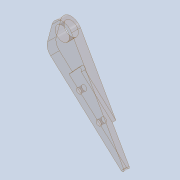
# Autodesk Inventor part: アーム先端
Saved by Autodesk Inventor 2020.4 (Build 244396000, 396)
## iProperties
Created: 2021-05-06
Part Number: アーム先端
Material: ポリカーボネート、スモーク
Document SubType Name: Modeling
Designer: happy
Density: 1.2 g/cm^3
Appearance: ポリカーボネート - スモーク
Author: happy
Autodesk Inventor part; units mm, degrees
ref_plane "YZ Plane" through (0, 0, 0) normal (1, 0, 0) x (0, 1, 0)
ref_plane "XZ Plane" through (0, 0, 0) normal (0, 1, 0) x (-1, 0, 0)
ref_plane "XY Plane" through (0, 0, 0) normal (0, 0, 1) x (1, 0, 0)
sketch "スケッチ1" plane through (0, 0, 0) normal (0, 0, 1) x (1, 0, 0)
  circle A0 centre (295.8489, -93.1201) radius 1.5
  circle A1 centre (295.8489, -93.1201) radius 3.025
  line L0 (302.9116, -92.7771) -> (291.3448, -101.5663)
  arc A2 (282.4058, -101.1768) -> (291.3448, -101.5663) centre (287.1097, -95.9928) ccw
  arc A3 (299.0788, -95.6895) -> (299.3467, -89.5424) centre (296.6588, -92.5047) ccw
  line L1 (214.4137, -12.4754) -> (302.9116, -92.7771)
  line L2 (186.8707, -14.4897) -> (289.472, -107.5885)
  line L3 (89.5137, -53) -> (377.0482, -53)
  circle A4 centre (295.8489, -93.1201) radius 4.025
  circle A5 centre (295.8489, -93.1201) radius 6
  line L4 (290.0522, -91.5712) -> (285.5936, -108.2576)
  circle A6 centre (285.4262, -97.1659) radius 3.025
  arc A7 (287.4387, -101.3525) -> (289.2034, -107.3448) centre (293.2353, -102.9014) ccw
  circle A8 centre (298.0159, -108.5895) radius 3
  circle A9 centre (298.0159, -108.5895) radius 1.5
  line L5 (185.1065, 0.6143) -> (481.3339, -268.178)
  line L6 (295.8489, -93.1201) -> (289.2034, -100.4438) construction
  line L7 (301.0696, -90.1631) -> (333.6375, -147.6637)
  line L8 (333.6375, -147.6637) -> (289.2034, -107.3448)
  circle A10 centre (295.8489, -93.1201) radius 1.5
  circle A11 centre (295.8489, -93.1201) radius 3.025
  line L9 (302.9116, -92.7771) -> (291.3448, -101.5663)
  arc A12 (282.4058, -101.1768) -> (291.3448, -101.5663) centre (287.1097, -95.9928) ccw
  arc A13 (299.0788, -95.6895) -> (299.3467, -89.5424) centre (296.6588, -92.5047) ccw
  line L10 (214.4137, -12.4754) -> (302.9116, -92.7771)
  line L11 (186.8707, -14.4897) -> (289.472, -107.5885)
  line L12 (89.5137, -53) -> (377.0482, -53)
  circle A14 centre (295.8489, -93.1201) radius 4.025
  circle A15 centre (295.8489, -93.1201) radius 6
  line L13 (290.0522, -91.5712) -> (285.5936, -108.2576)
  circle A16 centre (285.4262, -97.1659) radius 3.025
  arc A17 (287.4387, -101.3525) -> (289.2034, -107.3448) centre (293.2353, -102.9014) ccw
  circle A18 centre (298.0159, -108.5895) radius 3 construction
  circle A19 centre (298.0159, -108.5895) radius 1.5
  line L14 (185.1065, 0.6143) -> (481.3339, -268.178)
  line L15 (295.8489, -93.1201) -> (289.2034, -100.4438) construction
  line L16 (301.0696, -90.1631) -> (333.6375, -147.6637)
  line L17 (333.6375, -147.6637) -> (289.2034, -107.3448)
  line L18 (301.985, -108.1401) -> (343.1845, -145.5239)
  circle A20 centre (305.2216, -116.4782) radius 1.5
  circle A21 centre (316.3301, -126.5579) radius 1.5
  line L19 (301.985, -108.1401) -> (293.4984, -117.4928)
  arc A22 (303.5401, -109.5512) -> (301.985, -108.1401) centre (302.7625, -108.8456) ccw
  line L20 (301.985, -108.1401) -> (302.7625, -108.8456) construction
  line L21 (303.5401, -109.5512) -> (302.7625, -108.8456) construction
  point P0 (0, 0)
  point P1 (0, 0)
  point P2 (297.9123, -96.5759)
  point P3 (298.6256, -96.0339)
  point P4 (0, 0)
  point P5 (296.6091, -114.0646)
  point P6 (321.0497, -125.4392)
  dimension "d0" = 8.05
  dimension "d1" = 12
  dimension "d2" = 6
  dimension "d3" = 6
  dimension "d4" = 3
  dimension "d5" = 5
  dimension "d6" = 12
  dimension "d7" = 60
  dimension "d11" = 8.05
  dimension "d12" = 12
  dimension "d13" = 6
  dimension "d14" = 6
  dimension "d15" = 3
  dimension "d16" = 5
  dimension "d17" = 12
  dimension "d18" = 60
  dimension "d19" = 8
  dimension "d20" = 4
  dimension "d21" = 4
  dimension "d22" = 3
  dimension "d23" = 50
  dimension "d24" = 8
  dimension "d25" = 15
  dimension "d28" = 1.05
  dimension "d29" = 180
  constraints: 44 end point, 23 centre point, 18 point on circle, 13 tangent, 6 coincident, 6 point on line, 3 perpendicular, 1 equal radius, 12 other
  measures "d0" diameter of A4
  measures "d1" diameter of A5
  measures "d2" radius of A7
  measures "d3" diameter of A8
  measures "d4" diameter of A9
  measures "d5" distance from line of A9.centre L5
  measures "d6" distance from line of A8.centre L6
  measures "d7" distance of L7.end L8.end
  measures "d11" diameter of A14
  measures "d12" diameter of A15
  measures "d13" radius of A17
  measures "d14" diameter of A18
  measures "d15" diameter of A19
  measures "d16" distance from line of A19.centre L14
  measures "d17" distance from line of A18.centre L15
  measures "d18" distance of L16.end L17.end
  measures "d19" distance between parallel lines of L17 L18
  measures "d20" distance from line of L18 A20.centre
  measures "d21" distance from line of L18 A21.centre
  measures "d22" diameter of A20
  measures "d23" distance from line of L16.end L19
  measures "d24" distance from line of L19 A20.centre
  measures "d25" distance between centres of A21 A20
  measures "d28" radius of A22
  measures "d29" angle of L20 L21
extrude "押し出し1" add sketch "スケッチ1" along normal blind 5 contours L7 L5 A5 L0 | L0 A5 L1 L7 | L1 A5 L7 | A5 L5 L0 A4 | L0 A3 L1 A5 | L7 L18 A22 L19 A8 L8 L2 A7 A2 L0 A5 L5 | L1 A5 | L0 A4 L5 A5 L1 A3 | A5 L0 L5 | L7 L8 L19 A8 L18 | A4 L0 | A5 L5 L0 | L0 A2 A7 L4 L5 A5 | L18 A22 | A5 L5 L4 | L19 A8 | A8 L19 | A9 picked at (298.3132, -96.2806)
fillet "フィレット1" radius 1 1 edges at (333.6375, -147.6637, 2.5)
extrude "押し出し2" cut sketch "スケッチ1" along normal blind 2 contours L7 L8 L19 A8 L18 | L18 A22 | L19 A8 picked at (299.8706, -110.6044)
equation "\"d20\" = 0.5 * d19"
equation "\"d21\" = d20"
